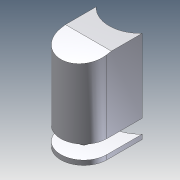
# Autodesk Inventor part: CANH TAY 1
Saved by Autodesk Inventor 2011 (Build 150239000, 239)
## iProperties
Manager: CÁI
Company: TPA
Created: 2018-05-23
Part Number: CANH TAY 1
Material: -
Document SubType Name: Modeling
Designer: hau.np
Surface Area: 1125.21 cm^2
Volume: 1704.41 cm^3
Author: hau.np
Comments: GHI CHÚ: 1. DUNG SAI KÍCH THƯỚC GIA CÔNG +/- 0.5 2. LÀM SẠCH BAVIA CẠNH CẮT. 3.
Autodesk Inventor part; units mm, degrees
ref_plane "YZ Plane" through (0, 0, 0) normal (1, 0, 0) x (0, 1, 0)
ref_plane "XZ Plane" through (0, 0, 0) normal (0, 1, 0) x (-1, 0, 0)
ref_plane "XY Plane" through (0, 0, 0) normal (0, 0, 1) x (1, 0, 0)
sketch "Sketch1" plane through (0, 0, 0) normal (0, 0, 1) x (1, 0, 0)
  line L0 (0, 15.9441) -> (0, -15.9441) construction
  line L1 (11.6084, 0) -> (-11.6084, 0) construction
  line L2 (50, 162.8204) -> (50, 85.9072)
  line L3 (50, 85.9072) -> (-50, 85.9072)
  line L4 (-50, 85.9072) -> (-50, 162.8204)
  circle A0 centre (0, 85.9072) radius 50
  arc A1 (-50, 162.8204) -> (50, 162.8204) centre (0, 208.9072) ccw
  point P0 (0, 0)
  point P1 (0, 0)
  point P2 (0, 165.9072)
  dimension "d5" = 100
  dimension "d7" = 136
  dimension "d8" = 123
  constraints: 10 end point, 3 midpoint, 2 point on circle, 1 centre point, 1 coincident, 1 horizontal, 1 horizontal alignment, 1 parallel, 1 point on line, 1 vertical, 3 other
  measures "d5" distance between parallel lines of L2 L4
  measures "d7" diameter of A1
  measures "d8" distance of point (0, 85.907) A1.centre
extrude "Extrusion1" add sketch "Sketch1" along normal blind 200
sketch "Sketch2" plane through (50, 85.9072, 0) normal (1, 0, 0) x (0, 0, -1)
  line L0 (-200, 10) -> (-186.1081, -68.7846)
  line L1 (-200, 10) -> (-200, -68.7846)
  line L2 (-200, -68.7846) -> (-186.1081, -68.7846)
  point P0 (0, -85.9072)
  constraints: 6 end point, 1 perpendicular
extrude "Extrusion2" cut sketch "Sketch2" against normal through all
sketch "Sketch3" plane through (50, 85.9072, 0) normal (1, 0, 0) x (0, 0, -1)
  line L0 (-40, 89.4296) -> (-10, 89.4296)
  line L1 (-10, 89.4296) -> (-10, -119.3946)
  line L2 (-10, -119.3946) -> (-40, -119.3946)
  line L3 (-40, -119.3946) -> (-40, 89.4296)
  line L4 (0, -50) -> (0, 0) projected
  line L5 (0, 76.9131) -> (-200, 76.9131) projected
  point P0 (0, -85.9072)
  dimension "d9" = 30
  dimension "d10" = 10
  constraints: 8 end point, 2 parallel, 1 horizontal, 1 perpendicular
  measures "d9" distance between parallel lines of L1 L3
  measures "d10" distance between parallel lines of L4 L1
extrude "Extrusion3" cut sketch "Sketch3" against normal through all
sketch "Sketch4" plane through (50, 85.9072, 10) normal (0, 0, 1) x (1, 0, 0)
  arc A0 (-100, 0) -> (0, 0) centre (-50, 0) ccw projected
  circle A1 centre (-50, 0) radius 10
  point P0 (-50, -85.9072)
  constraints: 1 centre point, 1 coincident
extrude "Extrusion4" add sketch "Sketch4" along normal blind 30
body "Solid1"
